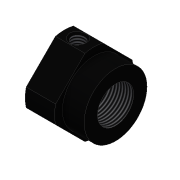
# Autodesk Inventor part: Wellenmutter
Saved by Autodesk Inventor 2016 (Build 200138000, 138)
## iProperties
Created: 2015-07-27
Part Number: Wellenmutter
Material: Steel
Document SubType Name: Modeling
Density: 7.85 g/cm^3
Appearance: Smooth - Black
Autodesk Inventor part; units mm, degrees
ref_plane "YZ Plane" through (0, 0, 0) normal (1, 0, 0) x (0, 1, 0)
ref_plane "XZ Plane" through (0, 0, 0) normal (0, 1, 0) x (-1, 0, 0)
ref_plane "XY Plane" through (0, 0, 0) normal (0, 0, 1) x (1, 0, 0)
sketch "Sketch1" plane through (0, 0, 0) normal (0, 0, 1) x (1, 0, 0)
  line L0 (0, 10) -> (0, 0)
  line L1 (0, 10) -> (7.5, 10)
  line L2 (7.5, 10) -> (7.5, 8)
  line L3 (7.5, 8) -> (13, 8)
  line L4 (13, 8) -> (13, 0)
  line L5 (13, 0) -> (0, 0)
  point P0 (0, 0)
  dimension "d0" = 16
  dimension "d1" = 20
  dimension "d2" = 13
  dimension "d3" = 7.5
  constraints: 12 end point, 4 perpendicular, 1 coincident, 1 horizontal, 1 vertical
  measures "d0" diameter of L3 L5
  measures "d1" diameter of L1 L5
  measures "d2" distance between parallel lines of L0 L4
  measures "d3" distance between parallel lines of L0 L2
revolve "Revolution1" add sketch "Sketch1" angle 360 about axis through (13, 0, 0) along (-1, 0, 0)
hole "Hole1" at (0, 0, 0) direction (1, 0, 0) diameter 9.188 end through all thread size "M10x0.75" class "6H" standard "ISO Metric profile"
sketch "Sketch2" plane through (0, 0, 0) normal (-1, 0, 0) x (0, 0, 1)
  line L0 (0, -12.0208) -> (12.0208, 0)
  line L1 (12.0208, 0) -> (0, 12.0208)
  line L2 (0, 12.0208) -> (-12.0208, 0)
  line L3 (-12.0208, 0) -> (0, -12.0208)
  line L4 (0, -12.0208) -> (0, 12.0208) construction
  line L5 (12.0208, 0) -> (-12.0208, 0) construction
  line L6 (0, -11.9) -> (0, 11.9) projected
  point P0 (0, 0)
  dimension "d14" = 17
  constraints: 12 end point, 4 perpendicular, 2 midpoint, 1 collinear
  measures "d14" distance of L1.end L2.end
extrude "Extrusion1" cut sketch "Sketch2" against normal through all keep common part
sketch "Sketch3" plane through (0, 0, 0) normal (0, 0, 1) x (1, 0, 0)
  line L0 (0, -2.2855) -> (0, 2.2855) projected
  point P0 (0, 0)
  point P1 (3.5, 0)
  point P2 (0, 0)
  dimension "d17" = 3.5
  constraints: 1 horizontal alignment, 1 midpoint
  measures "d17" distance from line of L0 point (3.5, 0)
hole "Hole2" at (3.5, 0, 0) direction (0, 0, 1) diameter 3.242 end through all thread size "M4x0.7" class "6H" standard "ISO Metric profile"
chamfer "Chamfer1" distance 0.5 angle 45 1 edges at (3.4896, -1.621, 9.8677)
body "Solid1"
